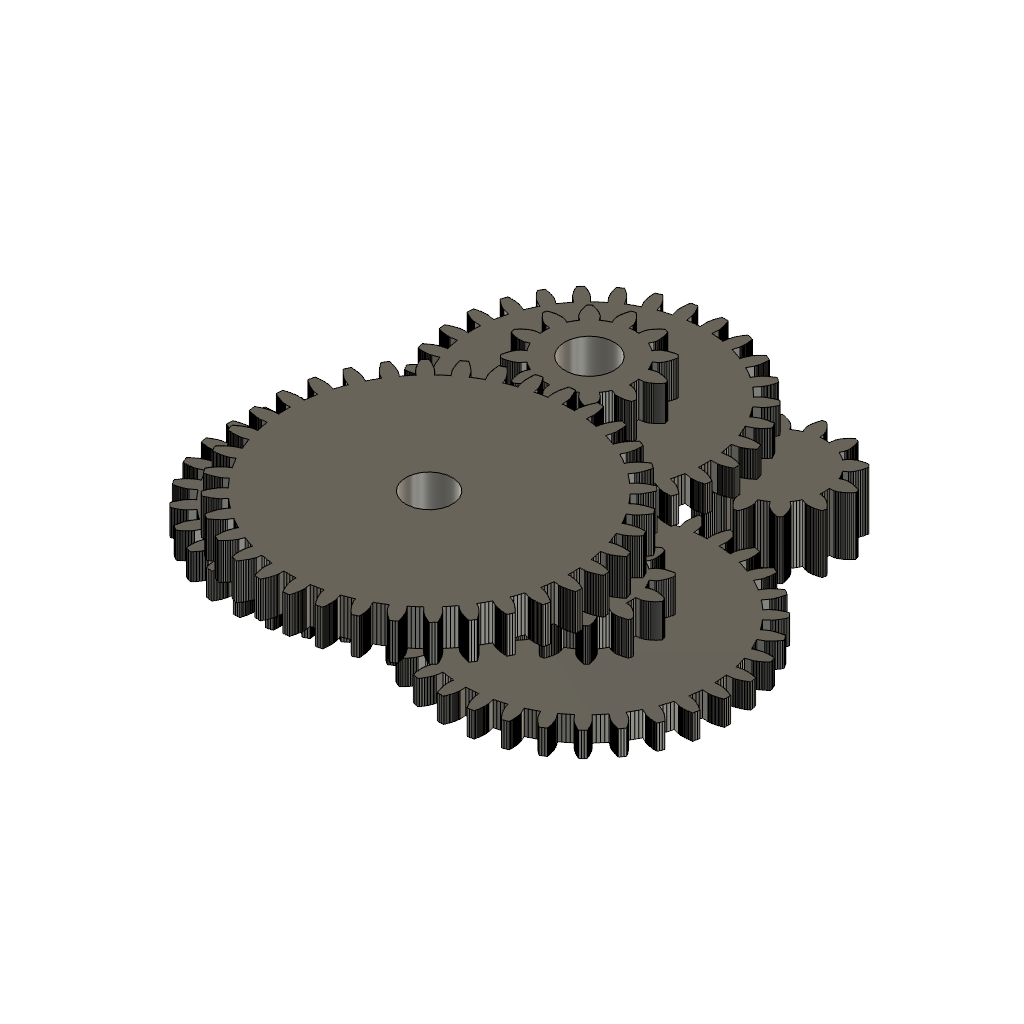
Infidex176V-IDENTIDEM.design-remix-counter-train (Autodesk Fusion 360 design; units mm, degrees)
part number: 2026-09-16-11-02-38-314
part number: 2026-09-27-15-41-25-852
part number: 2026-09-27-15-41-26-307
part number: 2026-09-27-15-41-28-841
part number: 2026-09-27-15-41-32-774
part number: 2026-09-27-15-41-37-132
Autodesk Fusion 360 part; units mm, degrees
(part 1 of 7)
ref_plane "WorkPlane1" through (0, 0, 36.8) normal (0, 0, 1) x (1, 0, 0) in component "CT sprocket pinion (tool body)"
sketch "Sketch1" plane through (0, 0, 36.8) normal (0, 0, 1) x (1, 0, 0) in component "CT sprocket pinion (tool body)"
  line L0 (76.2728, -44.8842) -> (76.564, -44.8534)
  line L1 (76.564, -44.8534) -> (76.6421, -44.8333)
  line L2 (76.6421, -44.8333) -> (76.719, -44.8033)
  line L3 (76.719, -44.8033) -> (76.7949, -44.7663)
  line L4 (76.7949, -44.7663) -> (76.8698, -44.7234)
  line L5 (76.8698, -44.7234) -> (76.9437, -44.6752)
  line L6 (76.9437, -44.6752) -> (77.0164, -44.622)
  line L7 (77.0164, -44.622) -> (77.0879, -44.5642)
  line L8 (77.0879, -44.5642) -> (77.1581, -44.5019)
  line L9 (77.1581, -44.5019) -> (77.2269, -44.4352)
  line L10 (77.2269, -44.4352) -> (77.2941, -44.3644)
  line L11 (77.2941, -44.3644) -> (77.3596, -44.2896)
  line L12 (77.3596, -44.2896) -> (77.4234, -44.2108)
  line L13 (77.4234, -44.2108) -> (77.403, -44.128)
  line L14 (77.403, -44.128) -> (77.3809, -44.0456)
  line L15 (77.3809, -44.0456) -> (77.3572, -43.9636)
  line L16 (77.3572, -43.9636) -> (77.2625, -43.9273)
  line L17 (77.2625, -43.9273) -> (77.1684, -43.8952)
  line L18 (77.1684, -43.8952) -> (77.0748, -43.8675)
  line L19 (77.0748, -43.8675) -> (76.9819, -43.8442)
  line L20 (76.9819, -43.8442) -> (76.89, -43.8253)
  line L21 (76.89, -43.8253) -> (76.7991, -43.811)
  line L22 (76.7991, -43.811) -> (76.7095, -43.8014)
  line L23 (76.7095, -43.8014) -> (76.6215, -43.7965)
  line L24 (76.6215, -43.7965) -> (76.5351, -43.7969)
  line L25 (76.5351, -43.7969) -> (76.4509, -43.8028)
  line L26 (76.4509, -43.8028) -> (76.3693, -43.8152)
  line L27 (76.3693, -43.8152) -> (76.2917, -43.8368)
  line L28 (76.2917, -43.8368) -> (76.024, -43.9557)
  line L29 (76.024, -43.9557) -> (75.9538, -43.8084)
  line L30 (75.9538, -43.8084) -> (75.876, -43.665)
  line L31 (75.876, -43.665) -> (75.7907, -43.5259)
  line L32 (75.7907, -43.5259) -> (75.6982, -43.3915)
  line L33 (75.6982, -43.3915) -> (75.935, -43.2191)
  line L34 (75.935, -43.2191) -> (75.9926, -43.1627)
  line L35 (75.9926, -43.1627) -> (76.0442, -43.0983)
  line L36 (76.0442, -43.0983) -> (76.0914, -43.0283)
  line L37 (76.0914, -43.0283) -> (76.1348, -42.9537)
  line L38 (76.1348, -42.9537) -> (76.1747, -42.875)
  line L39 (76.1747, -42.875) -> (76.2111, -42.7926)
  line L40 (76.2111, -42.7926) -> (76.2441, -42.7067)
  line L41 (76.2441, -42.7067) -> (76.2738, -42.6177)
  line L42 (76.2738, -42.6177) -> (76.3, -42.5256)
  line L43 (76.3, -42.5256) -> (76.3228, -42.4307)
  line L44 (76.3228, -42.4307) -> (76.3421, -42.3331)
  line L45 (76.3421, -42.3331) -> (76.358, -42.233)
  line L46 (76.358, -42.233) -> (76.2989, -42.1715)
  line L47 (76.2989, -42.1715) -> (76.2385, -42.1111)
  line L48 (76.2385, -42.1111) -> (76.177, -42.052)
  line L49 (76.177, -42.052) -> (76.0769, -42.0679)
  line L50 (76.0769, -42.0679) -> (75.9793, -42.0872)
  line L51 (75.9793, -42.0872) -> (75.8844, -42.11)
  line L52 (75.8844, -42.11) -> (75.7923, -42.1362)
  line L53 (75.7923, -42.1362) -> (75.7033, -42.1659)
  line L54 (75.7033, -42.1659) -> (75.6174, -42.1989)
  line L55 (75.6174, -42.1989) -> (75.535, -42.2353)
  line L56 (75.535, -42.2353) -> (75.4563, -42.2752)
  line L57 (75.4563, -42.2752) -> (75.3817, -42.3186)
  line L58 (75.3817, -42.3186) -> (75.3117, -42.3658)
  line L59 (75.3117, -42.3658) -> (75.2473, -42.4174)
  line L60 (75.2473, -42.4174) -> (75.1909, -42.475)
  line L61 (75.1909, -42.475) -> (75.0185, -42.7118)
  line L62 (75.0185, -42.7118) -> (74.8841, -42.6193)
  line L63 (74.8841, -42.6193) -> (74.745, -42.534)
  line L64 (74.745, -42.534) -> (74.6016, -42.4562)
  line L65 (74.6016, -42.4562) -> (74.4543, -42.386)
  line L66 (74.4543, -42.386) -> (74.5732, -42.1183)
  line L67 (74.5732, -42.1183) -> (74.5948, -42.0407)
  line L68 (74.5948, -42.0407) -> (74.6072, -41.9591)
  line L69 (74.6072, -41.9591) -> (74.6131, -41.8749)
  line L70 (74.6131, -41.8749) -> (74.6135, -41.7885)
  line L71 (74.6135, -41.7885) -> (74.6086, -41.7005)
  line L72 (74.6086, -41.7005) -> (74.599, -41.6109)
  line L73 (74.599, -41.6109) -> (74.5847, -41.52)
  line L74 (74.5847, -41.52) -> (74.5658, -41.4281)
  line L75 (74.5658, -41.4281) -> (74.5425, -41.3352)
  line L76 (74.5425, -41.3352) -> (74.5148, -41.2416)
  line L77 (74.5148, -41.2416) -> (74.4827, -41.1475)
  line L78 (74.4827, -41.1475) -> (74.4464, -41.0528)
  line L79 (74.4464, -41.0528) -> (74.3644, -41.0291)
  line L80 (74.3644, -41.0291) -> (74.282, -41.007)
  line L81 (74.282, -41.007) -> (74.1992, -40.9866)
  line L82 (74.1992, -40.9866) -> (74.1204, -41.0504)
  line L83 (74.1204, -41.0504) -> (74.0456, -41.1159)
  line L84 (74.0456, -41.1159) -> (73.9748, -41.1831)
  line L85 (73.9748, -41.1831) -> (73.9081, -41.2519)
  line L86 (73.9081, -41.2519) -> (73.8458, -41.3221)
  line L87 (73.8458, -41.3221) -> (73.788, -41.3936)
  line L88 (73.788, -41.3936) -> (73.7348, -41.4663)
  line L89 (73.7348, -41.4663) -> (73.6866, -41.5402)
  line L90 (73.6866, -41.5402) -> (73.6437, -41.6151)
  line L91 (73.6437, -41.6151) -> (73.6067, -41.691)
  line L92 (73.6067, -41.691) -> (73.5767, -41.7679)
  line L93 (73.5767, -41.7679) -> (73.5566, -41.846)
  line L94 (73.5566, -41.846) -> (73.5258, -42.1372)
  line L95 (73.5258, -42.1372) -> (73.3631, -42.1243)
  line L96 (73.3631, -42.1243) -> (73.2, -42.12)
  line L97 (73.2, -42.12) -> (73.0369, -42.1243)
  line L98 (73.0369, -42.1243) -> (72.8742, -42.1372)
  line L99 (72.8742, -42.1372) -> (72.8434, -41.846)
  line L100 (72.8434, -41.846) -> (72.8233, -41.7679)
  line L101 (72.8233, -41.7679) -> (72.7933, -41.691)
  line L102 (72.7933, -41.691) -> (72.7563, -41.6151)
  line L103 (72.7563, -41.6151) -> (72.7134, -41.5402)
  line L104 (72.7134, -41.5402) -> (72.6652, -41.4663)
  line L105 (72.6652, -41.4663) -> (72.612, -41.3936)
  line L106 (72.612, -41.3936) -> (72.5542, -41.3221)
  line L107 (72.5542, -41.3221) -> (72.4919, -41.2519)
  line L108 (72.4919, -41.2519) -> (72.4252, -41.1831)
  line L109 (72.4252, -41.1831) -> (72.3544, -41.1159)
  line L110 (72.3544, -41.1159) -> (72.2796, -41.0504)
  line L111 (72.2796, -41.0504) -> (72.2008, -40.9866)
  line L112 (72.2008, -40.9866) -> (72.118, -41.007)
  line L113 (72.118, -41.007) -> (72.0356, -41.0291)
  line L114 (72.0356, -41.0291) -> (71.9536, -41.0528)
  line L115 (71.9536, -41.0528) -> (71.9173, -41.1475)
  line L116 (71.9173, -41.1475) -> (71.8852, -41.2416)
  line L117 (71.8852, -41.2416) -> (71.8575, -41.3352)
  line L118 (71.8575, -41.3352) -> (71.8342, -41.4281)
  line L119 (71.8342, -41.4281) -> (71.8153, -41.52)
  line L120 (71.8153, -41.52) -> (71.801, -41.6109)
  line L121 (71.801, -41.6109) -> (71.7914, -41.7005)
  line L122 (71.7914, -41.7005) -> (71.7865, -41.7885)
  line L123 (71.7865, -41.7885) -> (71.7869, -41.8749)
  line L124 (71.7869, -41.8749) -> (71.7928, -41.9591)
  line L125 (71.7928, -41.9591) -> (71.8052, -42.0407)
  line L126 (71.8052, -42.0407) -> (71.8268, -42.1183)
  line L127 (71.8268, -42.1183) -> (71.9457, -42.386)
  line L128 (71.9457, -42.386) -> (71.7984, -42.4562)
  line L129 (71.7984, -42.4562) -> (71.655, -42.534)
  line L130 (71.655, -42.534) -> (71.5159, -42.6193)
  line L131 (71.5159, -42.6193) -> (71.3815, -42.7118)
  line L132 (71.3815, -42.7118) -> (71.2091, -42.475)
  line L133 (71.2091, -42.475) -> (71.1527, -42.4174)
  line L134 (71.1527, -42.4174) -> (71.0883, -42.3658)
  line L135 (71.0883, -42.3658) -> (71.0183, -42.3186)
  line L136 (71.0183, -42.3186) -> (70.9437, -42.2752)
  line L137 (70.9437, -42.2752) -> (70.865, -42.2353)
  line L138 (70.865, -42.2353) -> (70.7826, -42.1989)
  line L139 (70.7826, -42.1989) -> (70.6967, -42.1659)
  line L140 (70.6967, -42.1659) -> (70.6077, -42.1362)
  line L141 (70.6077, -42.1362) -> (70.5156, -42.11)
  line L142 (70.5156, -42.11) -> (70.4207, -42.0872)
  line L143 (70.4207, -42.0872) -> (70.3231, -42.0679)
  line L144 (70.3231, -42.0679) -> (70.223, -42.052)
  line L145 (70.223, -42.052) -> (70.1615, -42.1111)
  line L146 (70.1615, -42.1111) -> (70.1011, -42.1715)
  line L147 (70.1011, -42.1715) -> (70.042, -42.233)
  line L148 (70.042, -42.233) -> (70.0579, -42.3331)
  line L149 (70.0579, -42.3331) -> (70.0772, -42.4307)
  line L150 (70.0772, -42.4307) -> (70.1, -42.5256)
  line L151 (70.1, -42.5256) -> (70.1262, -42.6177)
  line L152 (70.1262, -42.6177) -> (70.1559, -42.7067)
  line L153 (70.1559, -42.7067) -> (70.1889, -42.7926)
  line L154 (70.1889, -42.7926) -> (70.2253, -42.875)
  line L155 (70.2253, -42.875) -> (70.2652, -42.9537)
  line L156 (70.2652, -42.9537) -> (70.3086, -43.0283)
  line L157 (70.3086, -43.0283) -> (70.3558, -43.0983)
  line L158 (70.3558, -43.0983) -> (70.4074, -43.1627)
  line L159 (70.4074, -43.1627) -> (70.465, -43.2191)
  line L160 (70.465, -43.2191) -> (70.7018, -43.3915)
  line L161 (70.7018, -43.3915) -> (70.6093, -43.5259)
  line L162 (70.6093, -43.5259) -> (70.524, -43.665)
  line L163 (70.524, -43.665) -> (70.4462, -43.8084)
  line L164 (70.4462, -43.8084) -> (70.376, -43.9557)
  line L165 (70.376, -43.9557) -> (70.1083, -43.8368)
  line L166 (70.1083, -43.8368) -> (70.0307, -43.8152)
  line L167 (70.0307, -43.8152) -> (69.9491, -43.8028)
  line L168 (69.9491, -43.8028) -> (69.8649, -43.7969)
  line L169 (69.8649, -43.7969) -> (69.7785, -43.7965)
  line L170 (69.7785, -43.7965) -> (69.6905, -43.8014)
  line L171 (69.6905, -43.8014) -> (69.6009, -43.811)
  line L172 (69.6009, -43.811) -> (69.51, -43.8253)
  line L173 (69.51, -43.8253) -> (69.4181, -43.8442)
  line L174 (69.4181, -43.8442) -> (69.3252, -43.8675)
  line L175 (69.3252, -43.8675) -> (69.2316, -43.8952)
  line L176 (69.2316, -43.8952) -> (69.1375, -43.9273)
  line L177 (69.1375, -43.9273) -> (69.0428, -43.9636)
  line L178 (69.0428, -43.9636) -> (69.0191, -44.0456)
  line L179 (69.0191, -44.0456) -> (68.997, -44.128)
  line L180 (68.997, -44.128) -> (68.9766, -44.2108)
  line L181 (68.9766, -44.2108) -> (69.0404, -44.2896)
  line L182 (69.0404, -44.2896) -> (69.1059, -44.3644)
  line L183 (69.1059, -44.3644) -> (69.1731, -44.4352)
  line L184 (69.1731, -44.4352) -> (69.2419, -44.5019)
  line L185 (69.2419, -44.5019) -> (69.3121, -44.5642)
  line L186 (69.3121, -44.5642) -> (69.3836, -44.622)
  line L187 (69.3836, -44.622) -> (69.4563, -44.6752)
  line L188 (69.4563, -44.6752) -> (69.5302, -44.7234)
  line L189 (69.5302, -44.7234) -> (69.6051, -44.7663)
  line L190 (69.6051, -44.7663) -> (69.681, -44.8033)
  line L191 (69.681, -44.8033) -> (69.7579, -44.8333)
  line L192 (69.7579, -44.8333) -> (69.836, -44.8534)
  line L193 (69.836, -44.8534) -> (70.1272, -44.8842)
  line L194 (70.1272, -44.8842) -> (70.1143, -45.0469)
  line L195 (70.1143, -45.0469) -> (70.11, -45.21)
  line L196 (70.11, -45.21) -> (70.1143, -45.3731)
  line L197 (70.1143, -45.3731) -> (70.1272, -45.5358)
  line L198 (70.1272, -45.5358) -> (69.836, -45.5666)
  line L199 (69.836, -45.5666) -> (69.7579, -45.5867)
  line L200 (69.7579, -45.5867) -> (69.681, -45.6167)
  line L201 (69.681, -45.6167) -> (69.6051, -45.6537)
  line L202 (69.6051, -45.6537) -> (69.5302, -45.6966)
  line L203 (69.5302, -45.6966) -> (69.4563, -45.7448)
  line L204 (69.4563, -45.7448) -> (69.3836, -45.798)
  line L205 (69.3836, -45.798) -> (69.3121, -45.8558)
  line L206 (69.3121, -45.8558) -> (69.2419, -45.9181)
  line L207 (69.2419, -45.9181) -> (69.1731, -45.9848)
  line L208 (69.1731, -45.9848) -> (69.1059, -46.0556)
  line L209 (69.1059, -46.0556) -> (69.0404, -46.1304)
  line L210 (69.0404, -46.1304) -> (68.9766, -46.2092)
  line L211 (68.9766, -46.2092) -> (68.997, -46.292)
  line L212 (68.997, -46.292) -> (69.0191, -46.3744)
  line L213 (69.0191, -46.3744) -> (69.0428, -46.4564)
  line L214 (69.0428, -46.4564) -> (69.1375, -46.4927)
  line L215 (69.1375, -46.4927) -> (69.2316, -46.5248)
  line L216 (69.2316, -46.5248) -> (69.3252, -46.5525)
  line L217 (69.3252, -46.5525) -> (69.4181, -46.5758)
  line L218 (69.4181, -46.5758) -> (69.51, -46.5947)
  line L219 (69.51, -46.5947) -> (69.6009, -46.609)
  line L220 (69.6009, -46.609) -> (69.6905, -46.6186)
  line L221 (69.6905, -46.6186) -> (69.7785, -46.6235)
  line L222 (69.7785, -46.6235) -> (69.8649, -46.6231)
  line L223 (69.8649, -46.6231) -> (69.9491, -46.6172)
  line L224 (69.9491, -46.6172) -> (70.0307, -46.6048)
  line L225 (70.0307, -46.6048) -> (70.1083, -46.5832)
  line L226 (70.1083, -46.5832) -> (70.376, -46.4643)
  line L227 (70.376, -46.4643) -> (70.4462, -46.6116)
  line L228 (70.4462, -46.6116) -> (70.524, -46.755)
  line L229 (70.524, -46.755) -> (70.6093, -46.8941)
  line L230 (70.6093, -46.8941) -> (70.7018, -47.0285)
  line L231 (70.7018, -47.0285) -> (70.465, -47.2009)
  line L232 (70.465, -47.2009) -> (70.4074, -47.2573)
  line L233 (70.4074, -47.2573) -> (70.3558, -47.3217)
  line L234 (70.3558, -47.3217) -> (70.3086, -47.3917)
  line L235 (70.3086, -47.3917) -> (70.2652, -47.4663)
  line L236 (70.2652, -47.4663) -> (70.2253, -47.545)
  line L237 (70.2253, -47.545) -> (70.1889, -47.6274)
  line L238 (70.1889, -47.6274) -> (70.1559, -47.7133)
  line L239 (70.1559, -47.7133) -> (70.1262, -47.8023)
  line L240 (70.1262, -47.8023) -> (70.1, -47.8944)
  line L241 (70.1, -47.8944) -> (70.0772, -47.9893)
  line L242 (70.0772, -47.9893) -> (70.0579, -48.0869)
  line L243 (70.0579, -48.0869) -> (70.042, -48.187)
  line L244 (70.042, -48.187) -> (70.1011, -48.2485)
  line L245 (70.1011, -48.2485) -> (70.1615, -48.3089)
  line L246 (70.1615, -48.3089) -> (70.223, -48.368)
  line L247 (70.223, -48.368) -> (70.3231, -48.3521)
  line L248 (70.3231, -48.3521) -> (70.4207, -48.3328)
  line L249 (70.4207, -48.3328) -> (70.5156, -48.31)
  line L250 (70.5156, -48.31) -> (70.6077, -48.2838)
  line L251 (70.6077, -48.2838) -> (70.6967, -48.2541)
  line L252 (70.6967, -48.2541) -> (70.7826, -48.2211)
  line L253 (70.7826, -48.2211) -> (70.865, -48.1847)
  line L254 (70.865, -48.1847) -> (70.9437, -48.1448)
  line L255 (70.9437, -48.1448) -> (71.0183, -48.1014)
  line L256 (71.0183, -48.1014) -> (71.0883, -48.0542)
  line L257 (71.0883, -48.0542) -> (71.1527, -48.0026)
  line L258 (71.1527, -48.0026) -> (71.2091, -47.945)
  line L259 (71.2091, -47.945) -> (71.3815, -47.7082)
  line L260 (71.3815, -47.7082) -> (71.5159, -47.8007)
  line L261 (71.5159, -47.8007) -> (71.655, -47.886)
  line L262 (71.655, -47.886) -> (71.7984, -47.9638)
  line L263 (71.7984, -47.9638) -> (71.9457, -48.034)
  line L264 (71.9457, -48.034) -> (71.8268, -48.3017)
  line L265 (71.8268, -48.3017) -> (71.8052, -48.3793)
  line L266 (71.8052, -48.3793) -> (71.7928, -48.4609)
  line L267 (71.7928, -48.4609) -> (71.7869, -48.5451)
  line L268 (71.7869, -48.5451) -> (71.7865, -48.6315)
  line L269 (71.7865, -48.6315) -> (71.7914, -48.7195)
  line L270 (71.7914, -48.7195) -> (71.801, -48.8091)
  line L271 (71.801, -48.8091) -> (71.8153, -48.9)
  line L272 (71.8153, -48.9) -> (71.8342, -48.9919)
  line L273 (71.8342, -48.9919) -> (71.8575, -49.0848)
  line L274 (71.8575, -49.0848) -> (71.8852, -49.1784)
  line L275 (71.8852, -49.1784) -> (71.9173, -49.2725)
  line L276 (71.9173, -49.2725) -> (71.9536, -49.3672)
  line L277 (71.9536, -49.3672) -> (72.0356, -49.3909)
  line L278 (72.0356, -49.3909) -> (72.118, -49.413)
  line L279 (72.118, -49.413) -> (72.2008, -49.4334)
  line L280 (72.2008, -49.4334) -> (72.2796, -49.3696)
  line L281 (72.2796, -49.3696) -> (72.3544, -49.3041)
  line L282 (72.3544, -49.3041) -> (72.4252, -49.2369)
  line L283 (72.4252, -49.2369) -> (72.4919, -49.1681)
  line L284 (72.4919, -49.1681) -> (72.5542, -49.0979)
  line L285 (72.5542, -49.0979) -> (72.612, -49.0264)
  line L286 (72.612, -49.0264) -> (72.6652, -48.9537)
  line L287 (72.6652, -48.9537) -> (72.7134, -48.8798)
  line L288 (72.7134, -48.8798) -> (72.7563, -48.8049)
  line L289 (72.7563, -48.8049) -> (72.7933, -48.729)
  line L290 (72.7933, -48.729) -> (72.8233, -48.6521)
  line L291 (72.8233, -48.6521) -> (72.8434, -48.574)
  line L292 (72.8434, -48.574) -> (72.8742, -48.2828)
  line L293 (72.8742, -48.2828) -> (73.0369, -48.2957)
  line L294 (73.0369, -48.2957) -> (73.2, -48.3)
  line L295 (73.2, -48.3) -> (73.3631, -48.2957)
  line L296 (73.3631, -48.2957) -> (73.5258, -48.2828)
  line L297 (73.5258, -48.2828) -> (73.5566, -48.574)
  line L298 (73.5566, -48.574) -> (73.5767, -48.6521)
  line L299 (73.5767, -48.6521) -> (73.6067, -48.729)
  line L300 (73.6067, -48.729) -> (73.6437, -48.8049)
  line L301 (73.6437, -48.8049) -> (73.6866, -48.8798)
  line L302 (73.6866, -48.8798) -> (73.7348, -48.9537)
  line L303 (73.7348, -48.9537) -> (73.788, -49.0264)
  line L304 (73.788, -49.0264) -> (73.8458, -49.0979)
  line L305 (73.8458, -49.0979) -> (73.9081, -49.1681)
  line L306 (73.9081, -49.1681) -> (73.9748, -49.2369)
  line L307 (73.9748, -49.2369) -> (74.0456, -49.3041)
  line L308 (74.0456, -49.3041) -> (74.1204, -49.3696)
  line L309 (74.1204, -49.3696) -> (74.1992, -49.4334)
  line L310 (74.1992, -49.4334) -> (74.282, -49.413)
  line L311 (74.282, -49.413) -> (74.3644, -49.3909)
  line L312 (74.3644, -49.3909) -> (74.4464, -49.3672)
  line L313 (74.4464, -49.3672) -> (74.4827, -49.2725)
  line L314 (74.4827, -49.2725) -> (74.5148, -49.1784)
  line L315 (74.5148, -49.1784) -> (74.5425, -49.0848)
  line L316 (74.5425, -49.0848) -> (74.5658, -48.9919)
  line L317 (74.5658, -48.9919) -> (74.5847, -48.9)
  line L318 (74.5847, -48.9) -> (74.599, -48.8091)
  line L319 (74.599, -48.8091) -> (74.6086, -48.7195)
  line L320 (74.6086, -48.7195) -> (74.6135, -48.6315)
  line L321 (74.6135, -48.6315) -> (74.6131, -48.5451)
  line L322 (74.6131, -48.5451) -> (74.6072, -48.4609)
  line L323 (74.6072, -48.4609) -> (74.5948, -48.3793)
  line L324 (74.5948, -48.3793) -> (74.5732, -48.3017)
  line L325 (74.5732, -48.3017) -> (74.4543, -48.034)
  line L326 (74.4543, -48.034) -> (74.6016, -47.9638)
  line L327 (74.6016, -47.9638) -> (74.745, -47.886)
  line L328 (74.745, -47.886) -> (74.8841, -47.8007)
  line L329 (74.8841, -47.8007) -> (75.0185, -47.7082)
  line L330 (75.0185, -47.7082) -> (75.1909, -47.945)
  line L331 (75.1909, -47.945) -> (75.2473, -48.0026)
  line L332 (75.2473, -48.0026) -> (75.3117, -48.0542)
  line L333 (75.3117, -48.0542) -> (75.3817, -48.1014)
  line L334 (75.3817, -48.1014) -> (75.4563, -48.1448)
  line L335 (75.4563, -48.1448) -> (75.535, -48.1847)
  line L336 (75.535, -48.1847) -> (75.6174, -48.2211)
  line L337 (75.6174, -48.2211) -> (75.7033, -48.2541)
  line L338 (75.7033, -48.2541) -> (75.7923, -48.2838)
  line L339 (75.7923, -48.2838) -> (75.8844, -48.31)
  line L340 (75.8844, -48.31) -> (75.9793, -48.3328)
  line L341 (75.9793, -48.3328) -> (76.0769, -48.3521)
  line L342 (76.0769, -48.3521) -> (76.177, -48.368)
  line L343 (76.177, -48.368) -> (76.2385, -48.3089)
  line L344 (76.2385, -48.3089) -> (76.2989, -48.2485)
  line L345 (76.2989, -48.2485) -> (76.358, -48.187)
  line L346 (76.358, -48.187) -> (76.3421, -48.0869)
  line L347 (76.3421, -48.0869) -> (76.3228, -47.9893)
  line L348 (76.3228, -47.9893) -> (76.3, -47.8944)
  line L349 (76.3, -47.8944) -> (76.2738, -47.8023)
  line L350 (76.2738, -47.8023) -> (76.2441, -47.7133)
  line L351 (76.2441, -47.7133) -> (76.2111, -47.6274)
  line L352 (76.2111, -47.6274) -> (76.1747, -47.545)
  line L353 (76.1747, -47.545) -> (76.1348, -47.4663)
  line L354 (76.1348, -47.4663) -> (76.0914, -47.3917)
  line L355 (76.0914, -47.3917) -> (76.0442, -47.3217)
  line L356 (76.0442, -47.3217) -> (75.9926, -47.2573)
  line L357 (75.9926, -47.2573) -> (75.935, -47.2009)
  line L358 (75.935, -47.2009) -> (75.6982, -47.0285)
  line L359 (75.6982, -47.0285) -> (75.7907, -46.8941)
  line L360 (75.7907, -46.8941) -> (75.876, -46.755)
  line L361 (75.876, -46.755) -> (75.9538, -46.6116)
  line L362 (75.9538, -46.6116) -> (76.024, -46.4643)
  line L363 (76.024, -46.4643) -> (76.2917, -46.5832)
  line L364 (76.2917, -46.5832) -> (76.3693, -46.6048)
  line L365 (76.3693, -46.6048) -> (76.4509, -46.6172)
  line L366 (76.4509, -46.6172) -> (76.5351, -46.6231)
  line L367 (76.5351, -46.6231) -> (76.6215, -46.6235)
  line L368 (76.6215, -46.6235) -> (76.7095, -46.6186)
  line L369 (76.7095, -46.6186) -> (76.7991, -46.609)
  line L370 (76.7991, -46.609) -> (76.89, -46.5947)
  line L371 (76.89, -46.5947) -> (76.9819, -46.5758)
  line L372 (76.9819, -46.5758) -> (77.0748, -46.5525)
  line L373 (77.0748, -46.5525) -> (77.1684, -46.5248)
  line L374 (77.1684, -46.5248) -> (77.2625, -46.4927)
  line L375 (77.2625, -46.4927) -> (77.3572, -46.4564)
  line L376 (77.3572, -46.4564) -> (77.3809, -46.3744)
  line L377 (77.3809, -46.3744) -> (77.403, -46.292)
  line L378 (77.403, -46.292) -> (77.4234, -46.2092)
  line L379 (77.4234, -46.2092) -> (77.3596, -46.1304)
  line L380 (77.3596, -46.1304) -> (77.2941, -46.0556)
  line L381 (77.2941, -46.0556) -> (77.2269, -45.9848)
  line L382 (77.2269, -45.9848) -> (77.1581, -45.9181)
  line L383 (77.1581, -45.9181) -> (77.0879, -45.8558)
  line L384 (77.0879, -45.8558) -> (77.0164, -45.798)
  line L385 (77.0164, -45.798) -> (76.9437, -45.7448)
  line L386 (76.9437, -45.7448) -> (76.8698, -45.6966)
  line L387 (76.8698, -45.6966) -> (76.7949, -45.6537)
  line L388 (76.7949, -45.6537) -> (76.719, -45.6167)
  line L389 (76.719, -45.6167) -> (76.6421, -45.5867)
  line L390 (76.6421, -45.5867) -> (76.564, -45.5666)
  line L391 (76.564, -45.5666) -> (76.2728, -45.5358)
  line L392 (76.2728, -45.5358) -> (76.2857, -45.3731)
  line L393 (76.2857, -45.3731) -> (76.29, -45.21)
  line L394 (76.29, -45.21) -> (76.2857, -45.0469)
  line L395 (76.2857, -45.0469) -> (76.2728, -44.8842)
extrude "Extrude1" add sketch "Sketch1" along normal blind 4 makes body 1 in component "CT sprocket pinion (tool body)"
ref_plane "WorkPlane1" through (0, 0, 36.8) normal (0, 0, 1) x (1, 0, 0) in component "CT idler 1"
sketch "Sketch1 (2)" plane through (0, 0, 36.8) normal (0, 0, 1) x (1, 0, 0) in component "CT idler 1"
  line L0 (78.2846, -51.5886) -> (78.5354, -51.263)
  line L1 (78.5354, -51.263) -> (78.576, -51.1997)
  line L2 (78.576, -51.1997) -> (78.6123, -51.1331)
  line L3 (78.6123, -51.1331) -> (78.6457, -51.0643)
  line L4 (78.6457, -51.0643) -> (78.6767, -50.9937)
  line L5 (78.6767, -50.9937) -> (78.7056, -50.9216)
  line L6 (78.7056, -50.9216) -> (78.7325, -50.848)
  line L7 (78.7325, -50.848) -> (78.7576, -50.7732)
  line L8 (78.7576, -50.7732) -> (78.781, -50.6971)
  line L9 (78.781, -50.6971) -> (78.8027, -50.6199)
  line L10 (78.8027, -50.6199) -> (78.8228, -50.5416)
  line L11 (78.8228, -50.5416) -> (78.8414, -50.4623)
  line L12 (78.8414, -50.4623) -> (78.8584, -50.3821)
  line L13 (78.8584, -50.3821) -> (78.744, -50.3002)
  line L14 (78.744, -50.3002) -> (78.6285, -50.22)
  line L15 (78.6285, -50.22) -> (78.5118, -50.1414)
  line L16 (78.5118, -50.1414) -> (78.4425, -50.1854)
  line L17 (78.4425, -50.1854) -> (78.3747, -50.2306)
  line L18 (78.3747, -50.2306) -> (78.3084, -50.2768)
  line L19 (78.3084, -50.2768) -> (78.2437, -50.3241)
  line L20 (78.2437, -50.3241) -> (78.1806, -50.3726)
  line L21 (78.1806, -50.3726) -> (78.1192, -50.4223)
  line L22 (78.1192, -50.4223) -> (78.0597, -50.4732)
  line L23 (78.0597, -50.4732) -> (78.0022, -50.5255)
  line L24 (78.0022, -50.5255) -> (77.9469, -50.5792)
  line L25 (77.9469, -50.5792) -> (77.8942, -50.6346)
  line L26 (77.8942, -50.6346) -> (77.8445, -50.6919)
  line L27 (77.8445, -50.6919) -> (77.7994, -50.752)
  line L28 (77.7994, -50.752) -> (77.582, -51.1009)
  line L29 (77.582, -51.1009) -> (77.4035, -50.9927)
  line L30 (77.4035, -50.9927) -> (77.2224, -50.8888)
  line L31 (77.2224, -50.8888) -> (77.0389, -50.7894)
  line L32 (77.0389, -50.7894) -> (76.853, -50.6944)
  line L33 (76.853, -50.6944) -> (77.0355, -50.3261)
  line L34 (77.0355, -50.3261) -> (77.063, -50.2561)
  line L35 (77.063, -50.2561) -> (77.0856, -50.1838)
  line L36 (77.0856, -50.1838) -> (77.1049, -50.1098)
  line L37 (77.1049, -50.1098) -> (77.1216, -50.0345)
  line L38 (77.1216, -50.0345) -> (77.1358, -49.9581)
  line L39 (77.1358, -49.9581) -> (77.1479, -49.8807)
  line L40 (77.1479, -49.8807) -> (77.1579, -49.8024)
  line L41 (77.1579, -49.8024) -> (77.166, -49.7232)
  line L42 (77.166, -49.7232) -> (77.1722, -49.6433)
  line L43 (77.1722, -49.6433) -> (77.1767, -49.5626)
  line L44 (77.1767, -49.5626) -> (77.1794, -49.4812)
  line L45 (77.1794, -49.4812) -> (77.1805, -49.3991)
  line L46 (77.1805, -49.3991) -> (77.0523, -49.3412)
  line L47 (77.0523, -49.3412) -> (76.9233, -49.285)
  line L48 (76.9233, -49.285) -> (76.7935, -49.2307)
  line L49 (76.7935, -49.2307) -> (76.7342, -49.2874)
  line L50 (76.7342, -49.2874) -> (76.6765, -49.3449)
  line L51 (76.6765, -49.3449) -> (76.6205, -49.4032)
  line L52 (76.6205, -49.4032) -> (76.5662, -49.4622)
  line L53 (76.5662, -49.4622) -> (76.5138, -49.5221)
  line L54 (76.5138, -49.5221) -> (76.4633, -49.5828)
  line L55 (76.4633, -49.5828) -> (76.4149, -49.6444)
  line L56 (76.4149, -49.6444) -> (76.3687, -49.7069)
  line L57 (76.3687, -49.7069) -> (76.325, -49.7703)
  line L58 (76.325, -49.7703) -> (76.284, -49.8349)
  line L59 (76.284, -49.8349) -> (76.2464, -49.9008)
  line L60 (76.2464, -49.9008) -> (76.2139, -49.9686)
  line L61 (76.2139, -49.9686) -> (76.0688, -50.3532)
  line L62 (76.0688, -50.3532) -> (75.8726, -50.2819)
  line L63 (75.8726, -50.2819) -> (75.6748, -50.2153)
  line L64 (75.6748, -50.2153) -> (75.4754, -50.1536)
  line L65 (75.4754, -50.1536) -> (75.2745, -50.0967)
  line L66 (75.2745, -50.0967) -> (75.3817, -49.6999)
  line L67 (75.3817, -49.6999) -> (75.395, -49.6259)
  line L68 (75.395, -49.6259) -> (75.403, -49.5505)
  line L69 (75.403, -49.5505) -> (75.4076, -49.4742)
  line L70 (75.4076, -49.4742) -> (75.4092, -49.3971)
  line L71 (75.4092, -49.3971) -> (75.4083, -49.3194)
  line L72 (75.4083, -49.3194) -> (75.405, -49.2411)
  line L73 (75.405, -49.2411) -> (75.3995, -49.1624)
  line L74 (75.3995, -49.1624) -> (75.392, -49.0831)
  line L75 (75.392, -49.0831) -> (75.3825, -49.0035)
  line L76 (75.3825, -49.0035) -> (75.3712, -48.9235)
  line L77 (75.3712, -48.9235) -> (75.358, -48.8431)
  line L78 (75.358, -48.8431) -> (75.343, -48.7624)
  line L79 (75.343, -48.7624) -> (75.206, -48.7306)
  line L80 (75.206, -48.7306) -> (75.0685, -48.7007)
  line L81 (75.0685, -48.7007) -> (74.9306, -48.6728)
  line L82 (74.9306, -48.6728) -> (74.8835, -48.74)
  line L83 (74.8835, -48.74) -> (74.8381, -48.8076)
  line L84 (74.8381, -48.8076) -> (74.7945, -48.8757)
  line L85 (74.7945, -48.8757) -> (74.7529, -48.9442)
  line L86 (74.7529, -48.9442) -> (74.7131, -49.0131)
  line L87 (74.7131, -49.0131) -> (74.6755, -49.0825)
  line L88 (74.6755, -49.0825) -> (74.64, -49.1523)
  line L89 (74.64, -49.1523) -> (74.6069, -49.2226)
  line L90 (74.6069, -49.2226) -> (74.5763, -49.2934)
  line L91 (74.5763, -49.2934) -> (74.5488, -49.3647)
  line L92 (74.5488, -49.3647) -> (74.5248, -49.4367)
  line L93 (74.5248, -49.4367) -> (74.5061, -49.5095)
  line L94 (74.5061, -49.5095) -> (74.4388, -49.915)
  line L95 (74.4388, -49.915) -> (74.2325, -49.8834)
  line L96 (74.2325, -49.8834) -> (74.0255, -49.8567)
  line L97 (74.0255, -49.8567) -> (73.8179, -49.8351)
  line L98 (73.8179, -49.8351) -> (73.6098, -49.8185)
  line L99 (73.6098, -49.8185) -> (73.6375, -49.4084)
  line L100 (73.6375, -49.4084) -> (73.6361, -49.3332)
  line L101 (73.6361, -49.3332) -> (73.6292, -49.2577)
  line L102 (73.6292, -49.2577) -> (73.6188, -49.1819)
  line L103 (73.6188, -49.1819) -> (73.6053, -49.106)
  line L104 (73.6053, -49.106) -> (73.5893, -49.03)
  line L105 (73.5893, -49.03) -> (73.5708, -48.9539)
  line L106 (73.5708, -48.9539) -> (73.5501, -48.8777)
  line L107 (73.5501, -48.8777) -> (73.5273, -48.8014)
  line L108 (73.5273, -48.8014) -> (73.5024, -48.7252)
  line L109 (73.5024, -48.7252) -> (73.4757, -48.6489)
  line L110 (73.4757, -48.6489) -> (73.447, -48.5727)
  line L111 (73.447, -48.5727) -> (73.4166, -48.4965)
  line L112 (73.4166, -48.4965) -> (73.276, -48.492)
  line L113 (73.276, -48.492) -> (73.1353, -48.4895)
  line L114 (73.1353, -48.4895) -> (72.9947, -48.489)
  line L115 (72.9947, -48.489) -> (72.9616, -48.564)
  line L116 (72.9616, -48.564) -> (72.9302, -48.6392)
  line L117 (72.9302, -48.6392) -> (72.9008, -48.7145)
  line L118 (72.9008, -48.7145) -> (72.8733, -48.7898)
  line L119 (72.8733, -48.7898) -> (72.8477, -48.8652)
  line L120 (72.8477, -48.8652) -> (72.8243, -48.9406)
  line L121 (72.8243, -48.9406) -> (72.8032, -49.016)
  line L122 (72.8032, -49.016) -> (72.7844, -49.0914)
  line L123 (72.7844, -49.0914) -> (72.7683, -49.1668)
  line L124 (72.7683, -49.1668) -> (72.7551, -49.2421)
  line L125 (72.7551, -49.2421) -> (72.7456, -49.3174)
  line L126 (72.7456, -49.3174) -> (72.7416, -49.3924)
  line L127 (72.7416, -49.3924) -> (72.7547, -49.8033)
  line L128 (72.7547, -49.8033) -> (72.5461, -49.8125)
  line L129 (72.5461, -49.8125) -> (72.3379, -49.8267)
  line L130 (72.3379, -49.8267) -> (72.13, -49.846)
  line L131 (72.13, -49.846) -> (71.9227, -49.8703)
  line L132 (71.9227, -49.8703) -> (71.8699, -49.4627)
  line L133 (71.8699, -49.4627) -> (71.8538, -49.3892)
  line L134 (71.8538, -49.3892) -> (71.8324, -49.3165)
  line L135 (71.8324, -49.3165) -> (71.8074, -49.2442)
  line L136 (71.8074, -49.2442) -> (71.7794, -49.1724)
  line L137 (71.7794, -49.1724) -> (71.7488, -49.101)
  line L138 (71.7488, -49.101) -> (71.7158, -49.0299)
  line L139 (71.7158, -49.0299) -> (71.6806, -48.9593)
  line L140 (71.6806, -48.9593) -> (71.6434, -48.8889)
  line L141 (71.6434, -48.8889) -> (71.6041, -48.819)
  line L142 (71.6041, -48.819) -> (71.563, -48.7494)
  line L143 (71.563, -48.7494) -> (71.5201, -48.6802)
  line L144 (71.5201, -48.6802) -> (71.4753, -48.6114)
  line L145 (71.4753, -48.6114) -> (71.3366, -48.6344)
  line L146 (71.3366, -48.6344) -> (71.1981, -48.6594)
  line L147 (71.1981, -48.6594) -> (71.0601, -48.6864)
  line L148 (71.0601, -48.6864) -> (71.0422, -48.7665)
  line L149 (71.0422, -48.7665) -> (71.0262, -48.8463)
  line L150 (71.0262, -48.8463) -> (71.012, -48.9259)
  line L151 (71.012, -48.9259) -> (70.9997, -49.0051)
  line L152 (70.9997, -49.0051) -> (70.9894, -49.084)
  line L153 (70.9894, -49.084) -> (70.9811, -49.1626)
  line L154 (70.9811, -49.1626) -> (70.9751, -49.2407)
  line L155 (70.9751, -49.2407) -> (70.9714, -49.3183)
  line L156 (70.9714, -49.3183) -> (70.9703, -49.3954)
  line L157 (70.9703, -49.3954) -> (70.9721, -49.4718)
  line L158 (70.9721, -49.4718) -> (70.9774, -49.5474)
  line L159 (70.9774, -49.5474) -> (70.9881, -49.6219)
  line L160 (70.9881, -49.6219) -> (71.0811, -50.0223)
  line L161 (71.0811, -50.0223) -> (70.8784, -50.072)
  line L162 (70.8784, -50.072) -> (70.6769, -50.1266)
  line L163 (70.6769, -50.1266) -> (70.4768, -50.186)
  line L164 (70.4768, -50.186) -> (70.2782, -50.2503)
  line L165 (70.2782, -50.2503) -> (70.1468, -49.8608)
  line L166 (70.1468, -49.8608) -> (70.1168, -49.7919)
  line L167 (70.1168, -49.7919) -> (70.0816, -49.7248)
  line L168 (70.0816, -49.7248) -> (70.0429, -49.6588)
  line L169 (70.0429, -49.6588) -> (70.0015, -49.5938)
  line L170 (70.0015, -49.5938) -> (69.9575, -49.5297)
  line L171 (69.9575, -49.5297) -> (69.9113, -49.4664)
  line L172 (69.9113, -49.4664) -> (69.863, -49.404)
  line L173 (69.863, -49.404) -> (69.8128, -49.3423)
  line L174 (69.8128, -49.3423) -> (69.7606, -49.2813)
  line L175 (69.7606, -49.2813) -> (69.7067, -49.2211)
  line L176 (69.7067, -49.2211) -> (69.6511, -49.1616)
  line L177 (69.6511, -49.1616) -> (69.5938, -49.1029)
  line L178 (69.5938, -49.1029) -> (69.4622, -49.1525)
  line L179 (69.4622, -49.1525) -> (69.3313, -49.204)
  line L180 (69.3313, -49.204) -> (69.2011, -49.2574)
  line L181 (69.2011, -49.2574) -> (69.1993, -49.3395)
  line L182 (69.1993, -49.3395) -> (69.1991, -49.4209)
  line L183 (69.1991, -49.4209) -> (69.2007, -49.5017)
  line L184 (69.2007, -49.5017) -> (69.2041, -49.5818)
  line L185 (69.2041, -49.5818) -> (69.2094, -49.6612)
  line L186 (69.2094, -49.6612) -> (69.2166, -49.7398)
  line L187 (69.2166, -49.7398) -> (69.2259, -49.8176)
  line L188 (69.2259, -49.8176) -> (69.2374, -49.8945)
  line L189 (69.2374, -49.8945) -> (69.2514, -49.9703)
  line L190 (69.2514, -49.9703) -> (69.2681, -50.0449)
  line L191 (69.2681, -50.0449) -> (69.2881, -50.1181)
  line L192 (69.2881, -50.1181) -> (69.313, -50.189)
  line L193 (69.313, -50.189) -> (69.4824, -50.5635)
  line L194 (69.4824, -50.5635) -> (69.2932, -50.6518)
  line L195 (69.2932, -50.6518) -> (69.1063, -50.7447)
  line L196 (69.1063, -50.7447) -> (68.9216, -50.842)
  line L197 (68.9216, -50.842) -> (68.7394, -50.9439)
  line L198 (68.7394, -50.9439) -> (68.5346, -50.5875)
  line L199 (68.5346, -50.5875) -> (68.4916, -50.5257)
  line L200 (68.4916, -50.5257) -> (68.444, -50.4667)
  line L201 (68.444, -50.4667) -> (68.3932, -50.4096)
  line L202 (68.3932, -50.4096) -> (68.3399, -50.3539)
  line L203 (68.3399, -50.3539) -> (68.2843, -50.2996)
  line L204 (68.2843, -50.2996) -> (68.2266, -50.2466)
  line L205 (68.2266, -50.2466) -> (68.1671, -50.1948)
  line L206 (68.1671, -50.1948) -> (68.1058, -50.1441)
  line L207 (68.1058, -50.1441) -> (68.0427, -50.0944)
  line L208 (68.0427, -50.0944) -> (67.9781, -50.0459)
  line L209 (67.9781, -50.0459) -> (67.912, -49.9984)
  line L210 (67.912, -49.9984) -> (67.8443, -49.9519)
  line L211 (67.8443, -49.9519) -> (67.7249, -50.0263)
  line L212 (67.7249, -50.0263) -> (67.6066, -50.1024)
  line L213 (67.6066, -50.1024) -> (67.4893, -50.1801)
  line L214 (67.4893, -50.1801) -> (67.5035, -50.261)
  line L215 (67.5035, -50.261) -> (67.5192, -50.3409)
  line L216 (67.5192, -50.3409) -> (67.5366, -50.4198)
  line L217 (67.5366, -50.4198) -> (67.5555, -50.4977)
  line L218 (67.5555, -50.4977) -> (67.5762, -50.5746)
  line L219 (67.5762, -50.5746) -> (67.5986, -50.6503)
  line L220 (67.5986, -50.6503) -> (67.6229, -50.7248)
  line L221 (67.6229, -50.7248) -> (67.6492, -50.7979)
  line L222 (67.6492, -50.7979) -> (67.6777, -50.8695)
  line L223 (67.6777, -50.8695) -> (67.7086, -50.9394)
  line L224 (67.7086, -50.9394) -> (67.7425, -51.0073)
  line L225 (67.7425, -51.0073) -> (67.7808, -51.072)
  line L226 (67.7808, -51.072) -> (68.02, -51.4063)
  line L227 (68.02, -51.4063) -> (67.8517, -51.5298)
  line L228 (67.8517, -51.5298) -> (67.6864, -51.6573)
  line L229 (67.6864, -51.6573) -> (67.5243, -51.7888)
  line L230 (67.5243, -51.7888) -> (67.3655, -51.9243)
  line L231 (67.3655, -51.9243) -> (67.0951, -51.6147)
  line L232 (67.0951, -51.6147) -> (67.0409, -51.5625)
  line L233 (67.0409, -51.5625) -> (66.9827, -51.5139)
  line L234 (66.9827, -51.5139) -> (66.9217, -51.4678)
  line L235 (66.9217, -51.4678) -> (66.8586, -51.4236)
  line L236 (66.8586, -51.4236) -> (66.7934, -51.3812)
  line L237 (66.7934, -51.3812) -> (66.7265, -51.3404)
  line L238 (66.7265, -51.3404) -> (66.658, -51.3012)
  line L239 (66.658, -51.3012) -> (66.588, -51.2634)
  line L240 (66.588, -51.2634) -> (66.5165, -51.2271)
  line L241 (66.5165, -51.2271) -> (66.4436, -51.1921)
  line L242 (66.4436, -51.1921) -> (66.3695, -51.1584)
  line L243 (66.3695, -51.1584) -> (66.2941, -51.126)
  line L244 (66.2941, -51.126) -> (66.1915, -51.2223)
  line L245 (66.1915, -51.2223) -> (66.0903, -51.32)
  line L246 (66.0903, -51.32) -> (65.9904, -51.4191)
  line L247 (65.9904, -51.4191) -> (66.0201, -51.4956)
  line L248 (66.0201, -51.4956) -> (66.0511, -51.5709)
  line L249 (66.0511, -51.5709) -> (66.0835, -51.6449)
  line L250 (66.0835, -51.6449) -> (66.1173, -51.7177)
  line L251 (66.1173, -51.7177) -> (66.1526, -51.789)
  line L252 (66.1526, -51.789) -> (66.1893, -51.8589)
  line L253 (66.1893, -51.8589) -> (66.2277, -51.9272)
  line L254 (66.2277, -51.9272) -> (66.2677, -51.9938)
  line L255 (66.2677, -51.9938) -> (66.3096, -52.0585)
  line L256 (66.3096, -52.0585) -> (66.3536, -52.121)
  line L257 (66.3536, -52.121) -> (66.4001, -52.181)
  line L258 (66.4001, -52.181) -> (66.4503, -52.2369)
  line L259 (66.4503, -52.2369) -> (66.7501, -52.5181)
  line L260 (66.7501, -52.5181) -> (66.6091, -52.6721)
  line L261 (66.6091, -52.6721) -> (66.4719, -52.8294)
  line L262 (66.4719, -52.8294) -> (66.3386, -52.9901)
  line L263 (66.3386, -52.9901) -> (66.2092, -53.1539)
  line L264 (66.2092, -53.1539) -> (65.8836, -52.903)
  line L265 (65.8836, -52.903) -> (65.8203, -52.8624)
  line L266 (65.8203, -52.8624) -> (65.7537, -52.8261)
  line L267 (65.7537, -52.8261) -> (65.6849, -52.7927)
  line L268 (65.6849, -52.7927) -> (65.6144, -52.7617)
  line L269 (65.6144, -52.7617) -> (65.5422, -52.7328)
  line L270 (65.5422, -52.7328) -> (65.4687, -52.7059)
  line L271 (65.4687, -52.7059) -> (65.3938, -52.6808)
  line L272 (65.3938, -52.6808) -> (65.3177, -52.6574)
  line L273 (65.3177, -52.6574) -> (65.2405, -52.6357)
  line L274 (65.2405, -52.6357) -> (65.1623, -52.6156)
  line L275 (65.1623, -52.6156) -> (65.083, -52.597)
  line L276 (65.083, -52.597) -> (65.0027, -52.58)
  line L277 (65.0027, -52.58) -> (64.9208, -52.6944)
  line L278 (64.9208, -52.6944) -> (64.8406, -52.81)
  line L279 (64.8406, -52.81) -> (64.762, -52.9267)
  line L280 (64.762, -52.9267) -> (64.8061, -52.9959)
  line L281 (64.8061, -52.9959) -> (64.8512, -53.0637)
  line L282 (64.8512, -53.0637) -> (64.8974, -53.13)
  line L283 (64.8974, -53.13) -> (64.9447, -53.1948)
  line L284 (64.9447, -53.1948) -> (64.9932, -53.2578)
  line L285 (64.9932, -53.2578) -> (65.0429, -53.3192)
  line L286 (65.0429, -53.3192) -> (65.0939, -53.3787)
  line L287 (65.0939, -53.3787) -> (65.1461, -53.4362)
  line L288 (65.1461, -53.4362) -> (65.1999, -53.4915)
  line L289 (65.1999, -53.4915) -> (65.2552, -53.5442)
  line L290 (65.2552, -53.5442) -> (65.3125, -53.594)
  line L291 (65.3125, -53.594) -> (65.3726, -53.6391)
  line L292 (65.3726, -53.6391) -> (65.7215, -53.8564)
  line L293 (65.7215, -53.8564) -> (65.6133, -54.0349)
  line L294 (65.6133, -54.0349) -> (65.5095, -54.216)
  line L295 (65.5095, -54.216) -> (65.41, -54.3995)
  line L296 (65.41, -54.3995) -> (65.3151, -54.5854)
  line L297 (65.3151, -54.5854) -> (64.9468, -54.4029)
  line L298 (64.9468, -54.4029) -> (64.8768, -54.3754)
  line L299 (64.8768, -54.3754) -> (64.8044, -54.3528)
  line L300 (64.8044, -54.3528) -> (64.7304, -54.3335)
  line L301 (64.7304, -54.3335) -> (64.6551, -54.3168)
  line L302 (64.6551, -54.3168) -> (64.5787, -54.3026)
  line L303 (64.5787, -54.3026) -> (64.5013, -54.2905)
  line L304 (64.5013, -54.2905) -> (64.423, -54.2805)
  line L305 (64.423, -54.2805) -> (64.3439, -54.2724)
  line L306 (64.3439, -54.2724) -> (64.2639, -54.2662)
  line L307 (64.2639, -54.2662) -> (64.1832, -54.2617)
  line L308 (64.1832, -54.2617) -> (64.1018, -54.259)
  line L309 (64.1018, -54.259) -> (64.0197, -54.258)
  line L310 (64.0197, -54.258) -> (63.9618, -54.3861)
  line L311 (63.9618, -54.3861) -> (63.9057, -54.5151)
  line L312 (63.9057, -54.5151) -> (63.8514, -54.6449)
  line L313 (63.8514, -54.6449) -> (63.9081, -54.7042)
  line L314 (63.9081, -54.7042) -> (63.9655, -54.7619)
  line L315 (63.9655, -54.7619) -> (64.0238, -54.8179)
  line L316 (64.0238, -54.8179) -> (64.0829, -54.8722)
  line L317 (64.0829, -54.8722) -> (64.1427, -54.9246)
  line L318 (64.1427, -54.9246) -> (64.2034, -54.9751)
  line L319 (64.2034, -54.9751) -> (64.265, -55.0235)
  line L320 (64.265, -55.0235) -> (64.3275, -55.0697)
  line L321 (64.3275, -55.0697) -> (64.391, -55.1135)
  line L322 (64.391, -55.1135) -> (64.4555, -55.1544)
  line L323 (64.4555, -55.1544) -> (64.5214, -55.192)
  line L324 (64.5214, -55.192) -> (64.5892, -55.2245)
  line L325 (64.5892, -55.2245) -> (64.9738, -55.3696)
  line L326 (64.9738, -55.3696) -> (64.9025, -55.5658)
  line L327 (64.9025, -55.5658) -> (64.8359, -55.7636)
  line L328 (64.8359, -55.7636) -> (64.7742, -55.963)
  line L329 (64.7742, -55.963) -> (64.7174, -56.1639)
  line L330 (64.7174, -56.1639) -> (64.3205, -56.0567)
  line L331 (64.3205, -56.0567) -> (64.2465, -56.0434)
  line L332 (64.2465, -56.0434) -> (64.1711, -56.0354)
  line L333 (64.1711, -56.0354) -> (64.0948, -56.0309)
  line L334 (64.0948, -56.0309) -> (64.0177, -56.0292)
  line L335 (64.0177, -56.0292) -> (63.94, -56.0302)
  line L336 (63.94, -56.0302) -> (63.8617, -56.0334)
  line L337 (63.8617, -56.0334) -> (63.783, -56.0389)
  line L338 (63.783, -56.0389) -> (63.7038, -56.0464)
  line L339 (63.7038, -56.0464) -> (63.6241, -56.0559)
  line L340 (63.6241, -56.0559) -> (63.5441, -56.0673)
  line L341 (63.5441, -56.0673) -> (63.4637, -56.0805)
  line L342 (63.4637, -56.0805) -> (63.3831, -56.0954)
  line L343 (63.3831, -56.0954) -> (63.3512, -56.2325)
  line L344 (63.3512, -56.2325) -> (63.3213, -56.3699)
  line L345 (63.3213, -56.3699) -> (63.2934, -56.5078)
  line L346 (63.2934, -56.5078) -> (63.3606, -56.5549)
  line L347 (63.3606, -56.5549) -> (63.4282, -56.6003)
  line L348 (63.4282, -56.6003) -> (63.4963, -56.6439)
  line L349 (63.4963, -56.6439) -> (63.5648, -56.6856)
  line L350 (63.5648, -56.6856) -> (63.6337, -56.7253)
  line L351 (63.6337, -56.7253) -> (63.7031, -56.763)
  line L352 (63.7031, -56.763) -> (63.773, -56.7984)
  line L353 (63.773, -56.7984) -> (63.8433, -56.8316)
  line L354 (63.8433, -56.8316) -> (63.914, -56.8621)
  line L355 (63.914, -56.8621) -> (63.9854, -56.8897)
  line L356 (63.9854, -56.8897) -> (64.0573, -56.9137)
  line L357 (64.0573, -56.9137) -> (64.1301, -56.9323)
  line L358 (64.1301, -56.9323) -> (64.5356, -56.9996)
  line L359 (64.5356, -56.9996) -> (64.504, -57.2059)
  line L360 (64.504, -57.2059) -> (64.4773, -57.4129)
  line L361 (64.4773, -57.4129) -> (64.4557, -57.6206)
  line L362 (64.4557, -57.6206) -> (64.4391, -57.8287)
  line L363 (64.4391, -57.8287) -> (64.029, -57.801)
  line L364 (64.029, -57.801) -> (63.9538, -57.8024)
  line L365 (63.9538, -57.8024) -> (63.8783, -57.8092)
  line L366 (63.8783, -57.8092) -> (63.8025, -57.8196)
  line L367 (63.8025, -57.8196) -> (63.7266, -57.8331)
  line L368 (63.7266, -57.8331) -> (63.6506, -57.8491)
  line L369 (63.6506, -57.8491) -> (63.5745, -57.8676)
  line L370 (63.5745, -57.8676) -> (63.4983, -57.8883)
  line L371 (63.4983, -57.8883) -> (63.4221, -57.9112)
  line L372 (63.4221, -57.9112) -> (63.3458, -57.936)
  line L373 (63.3458, -57.936) -> (63.2695, -57.9628)
  line L374 (63.2695, -57.9628) -> (63.1933, -57.9914)
  line L375 (63.1933, -57.9914) -> (63.1171, -58.0218)
  line L376 (63.1171, -58.0218) -> (63.1126, -58.1624)
  line L377 (63.1126, -58.1624) -> (63.1101, -58.3031)
  line L378 (63.1101, -58.3031) -> (63.1096, -58.4437)
  line L379 (63.1096, -58.4437) -> (63.1847, -58.4769)
  line L380 (63.1847, -58.4769) -> (63.2599, -58.5082)
  line L381 (63.2599, -58.5082) -> (63.3351, -58.5376)
  line L382 (63.3351, -58.5376) -> (63.4104, -58.5652)
  line L383 (63.4104, -58.5652) -> (63.4858, -58.5907)
  line L384 (63.4858, -58.5907) -> (63.5612, -58.6141)
  line L385 (63.5612, -58.6141) -> (63.6366, -58.6353)
  line L386 (63.6366, -58.6353) -> (63.712, -58.654)
  line L387 (63.712, -58.654) -> (63.7874, -58.6701)
  line L388 (63.7874, -58.6701) -> (63.8628, -58.6833)
  line L389 (63.8628, -58.6833) -> (63.938, -58.6928)
  line L390 (63.938, -58.6928) -> (64.0131, -58.6969)
  line L391 (64.0131, -58.6969) -> (64.4239, -58.6837)
  line L392 (64.4239, -58.6837) -> (64.4331, -58.8923)
  line L393 (64.4331, -58.8923) -> (64.4473, -59.1005)
  line L394 (64.4473, -59.1005) -> (64.4666, -59.3084)
  line L395 (64.4666, -59.3084) -> (64.491, -59.5157)
  line L396 (64.491, -59.5157) -> (64.0833, -59.5686)
  line L397 (64.0833, -59.5686) -> (64.0099, -59.5846)
  line L398 (64.0099, -59.5846) -> (63.9371, -59.606)
  line L399 (63.9371, -59.606) -> (63.8649, -59.6311)
  line L400 (63.8649, -59.6311) -> (63.793, -59.659)
  line L401 (63.793, -59.659) -> (63.7216, -59.6896)
  line L402 (63.7216, -59.6896) -> (63.6506, -59.7226)
  line L403 (63.6506, -59.7226) -> (63.5799, -59.7578)
  line L404 (63.5799, -59.7578) -> (63.5096, -59.7951)
  line L405 (63.5096, -59.7951) -> (63.4396, -59.8343)
  line L406 (63.4396, -59.8343) -> (63.37, -59.8754)
  line L407 (63.37, -59.8754) -> (63.3008, -59.9184)
  line L408 (63.3008, -59.9184) -> (63.232, -59.9631)
  line L409 (63.232, -59.9631) -> (63.255, -60.1019)
  line L410 (63.255, -60.1019) -> (63.28, -60.2403)
  line L411 (63.28, -60.2403) -> (63.307, -60.3784)
  line L412 (63.307, -60.3784) -> (63.3871, -60.3962)
  line L413 (63.3871, -60.3962) -> (63.4669, -60.4122)
  line L414 (63.4669, -60.4122) -> (63.5465, -60.4264)
  line L415 (63.5465, -60.4264) -> (63.6258, -60.4387)
  line L416 (63.6258, -60.4387) -> (63.7047, -60.4491)
  line L417 (63.7047, -60.4491) -> (63.7832, -60.4573)
  line L418 (63.7832, -60.4573) -> (63.8613, -60.4634)
  line L419 (63.8613, -60.4634) -> (63.9389, -60.4671)
  line L420 (63.9389, -60.4671) -> (64.016, -60.4682)
  line L421 (64.016, -60.4682) -> (64.0924, -60.4663)
  line L422 (64.0924, -60.4663) -> (64.1681, -60.461)
  line L423 (64.1681, -60.461) -> (64.2425, -60.4503)
  line L424 (64.2425, -60.4503) -> (64.6429, -60.3573)
  line L425 (64.6429, -60.3573) -> (64.6926, -60.5601)
  line L426 (64.6926, -60.5601) -> (64.7472, -60.7615)
  line L427 (64.7472, -60.7615) -> (64.8067, -60.9616)
  line L428 (64.8067, -60.9616) -> (64.871, -61.1602)
  line L429 (64.871, -61.1602) -> (64.4815, -61.2916)
  line L430 (64.4815, -61.2916) -> (64.4125, -61.3217)
  line L431 (64.4125, -61.3217) -> (64.3454, -61.3569)
  line L432 (64.3454, -61.3569) -> (64.2794, -61.3955)
  line L433 (64.2794, -61.3955) -> (64.2144, -61.437)
  line L434 (64.2144, -61.437) -> (64.1503, -61.4809)
  line L435 (64.1503, -61.4809) -> (64.0871, -61.5271)
  line L436 (64.0871, -61.5271) -> (64.0246, -61.5754)
  line L437 (64.0246, -61.5754) -> (63.9629, -61.6257)
  line L438 (63.9629, -61.6257) -> (63.902, -61.6778)
  line L439 (63.902, -61.6778) -> (63.8417, -61.7317)
  line L440 (63.8417, -61.7317) -> (63.7823, -61.7873)
  line L441 (63.7823, -61.7873) -> (63.7235, -61.8446)
  line L442 (63.7235, -61.8446) -> (63.7731, -61.9762)
  line L443 (63.7731, -61.9762) -> (63.8247, -62.1071)
  line L444 (63.8247, -62.1071) -> (63.878, -62.2373)
  line L445 (63.878, -62.2373) -> (63.9601, -62.2392)
  line L446 (63.9601, -62.2392) -> (64.0415, -62.2393)
  line L447 (64.0415, -62.2393) -> (64.1223, -62.2377)
  line L448 (64.1223, -62.2377) -> (64.2024, -62.2343)
  line L449 (64.2024, -62.2343) -> (64.2818, -62.2291)
  line L450 (64.2818, -62.2291) -> (64.3605, -62.2218)
  line L451 (64.3605, -62.2218) -> (64.4382, -62.2125)
  line L452 (64.4382, -62.2125) -> (64.5151, -62.201)
  line L453 (64.5151, -62.201) -> (64.5909, -62.1871)
  line L454 (64.5909, -62.1871) -> (64.6655, -62.1704)
  line L455 (64.6655, -62.1704) -> (64.7387, -62.1503)
  line L456 (64.7387, -62.1503) -> (64.8096, -62.1254)
  line L457 (64.8096, -62.1254) -> (65.1841, -61.956)
  line L458 (65.1841, -61.956) -> (65.2724, -62.1452)
  line L459 (65.2724, -62.1452) -> (65.3653, -62.3321)
  line L460 (65.3653, -62.3321) -> (65.4627, -62.5168)
  line L461 (65.4627, -62.5168) -> (65.5645, -62.699)
  line L462 (65.5645, -62.699) -> (65.2081, -62.9038)
  line L463 (65.2081, -62.9038) -> (65.1464, -62.9468)
  line L464 (65.1464, -62.9468) -> (65.0874, -62.9944)
  line L465 (65.0874, -62.9944) -> (65.0302, -63.0452)
  line L466 (65.0302, -63.0452) -> (64.9745, -63.0985)
  line L467 (64.9745, -63.0985) -> (64.9203, -63.1541)
  line L468 (64.9203, -63.1541) -> (64.8672, -63.2118)
  line L469 (64.8672, -63.2118) -> (64.8154, -63.2713)
  line L470 (64.8154, -63.2713) -> (64.7647, -63.3327)
  line L471 (64.7647, -63.3327) -> (64.7151, -63.3957)
  line L472 (64.7151, -63.3957) -> (64.6665, -63.4603)
  line L473 (64.6665, -63.4603) -> (64.619, -63.5265)
  line L474 (64.619, -63.5265) -> (64.5726, -63.5941)
  line L475 (64.5726, -63.5941) -> (64.647, -63.7135)
  line L476 (64.647, -63.7135) -> (64.723, -63.8319)
  line L477 (64.723, -63.8319) -> (64.8008, -63.9491)
  line L478 (64.8008, -63.9491) -> (64.8816, -63.9349)
  line L479 (64.8816, -63.9349) -> (64.9615, -63.9192)
  line L480 (64.9615, -63.9192) -> (65.0404, -63.9019)
  line L481 (65.0404, -63.9019) -> (65.1184, -63.8829)
  line L482 (65.1184, -63.8829) -> (65.1952, -63.8622)
  line L483 (65.1952, -63.8622) -> (65.2709, -63.8398)
  line L484 (65.2709, -63.8398) -> (65.3454, -63.8155)
  line L485 (65.3454, -63.8155) -> (65.4185, -63.7892)
  line L486 (65.4185, -63.7892) -> (65.4901, -63.7607)
  line L487 (65.4901, -63.7607) -> (65.5601, -63.7298)
  line L488 (65.5601, -63.7298) -> (65.6279, -63.6959)
  line L489 (65.6279, -63.6959) -> (65.6926, -63.6576)
  line L490 (65.6926, -63.6576) -> (66.0269, -63.4184)
  line L491 (66.0269, -63.4184) -> (66.1504, -63.5867)
  line L492 (66.1504, -63.5867) -> (66.278, -63.752)
  line L493 (66.278, -63.752) -> (66.4095, -63.9141)
  line L494 (66.4095, -63.9141) -> (66.5449, -64.073)
  line L495 (66.5449, -64.073) -> (66.2353, -64.3434)
  line L496 (66.2353, -64.3434) -> (66.1831, -64.3975)
  line L497 (66.1831, -64.3975) -> (66.1346, -64.4557)
  line L498 (66.1346, -64.4557) -> (66.0884, -64.5167)
  line L499 (66.0884, -64.5167) -> (66.0442, -64.5799)
  line L500 (66.0442, -64.5799) -> (66.0018, -64.645)
  line L501 (66.0018, -64.645) -> (65.9611, -64.7119)
  line L502 (65.9611, -64.7119) -> (65.9218, -64.7804)
  line L503 (65.9218, -64.7804) -> (65.8841, -64.8505)
  line L504 (65.8841, -64.8505) -> (65.8477, -64.9219)
  line L505 (65.8477, -64.9219) -> (65.8127, -64.9948)
  line L506 (65.8127, -64.9948) -> (65.779, -65.0689)
  line L507 (65.779, -65.0689) -> (65.7467, -65.1443)
  line L508 (65.7467, -65.1443) -> (65.8429, -65.2469)